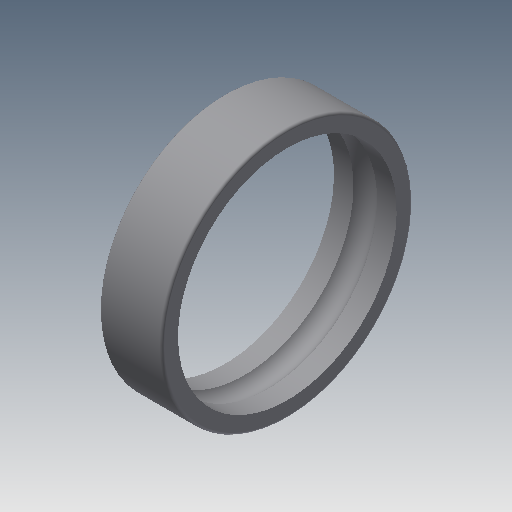
# Autodesk Inventor part: 676A Outer ring
Saved by Autodesk Inventor 2019.4 (Build 234330000, 330)
## iProperties
Category: PARTsolutions
Company: NTN
Created: 2019-06-11
Part Number: 676A Outer ring
Material: 一般
Catalog Web Link: www.cadenas.de
Description: Six types or-Metric system sizes
Vendor: NTN
Document SubType Name: Modeling
Designer: psadmin
Manufacturer: NTN
Mass: 0.0426535 g
Surface Area: 1.86998 cm^2
Volume: 0.0426535 cm^3
Density: 1 g/cm^3
Appearance: PSOLRGB-192-192-192
PSOL_IDENT_0: {$CADENAS_DATA\23d-libs\ntn\ball_roller_bearings\miniature_extra_small_bb\metric_system_sizes\mss_or
PSOL_IDENT_1: .prj},178 {VTYP=3D},{NB=676A Outer ring},{LINA=676A Outer ring},{NN=Six types or},{DATE=29.01.2019 2
PSOL_IDENT_2: 3:03:33},{GEOMDATE=02.04.2007 00:00:00},{VERSION=},{LINEID=9710},{WBVAR=},{WBNUMERIC=}  {NB=676A Out
PSOL_IDENT_3: er ring},{LINA=676A Outer ring},{KT=DUMMY},{IDNR=},{SD=6.0},{D=10},{B=2.5},{R=0.10},{ORDER=676A},{CR=
PSOL_IDENT_4: 465},{COR=196},{CRF=47},{CORF=20},{LSG=43 000},{LSO=51 000},{MASS=0.65},{D1=11.2},{D2=11.2},{C1=0.6}
PSOL_IDENT_5: ,{C2=0.6},{ORDER1=676A},{WSS=WA676AZ},{WDS=ZZ},{UTWF=FL676A},{FORSS=FLWA676AZ},{FORDS=ZZ},{DA1=6,6},
PSOL_IDENT_6: {DA2=6,7},{DA=9,2},{RAS=0,1},{MASS1=0.74},{B1=3.0},{VERS=1},{X=2},{N=12},{O=25.12},{RB=0.592}
NN: Six types or
NT: Metric system sizes
NB: 676A Outer ring
NBSYN: $ORDER. Outer ring
LINA: 676A Outer ring
SD: 6
D: 10
B: 2.5
R: 0.1
CR: 465
COR: 196
CRF: 47
CORF: 20
LSG: 43 000
LSO: 51 000
MASS: 0.65
D1: 11.2
D2: 11.2
C1: 0.6
C2: 0.6
ORDER1: 676A
WSS: WA676AZ
WDS: ZZ
UTWF: FL676A
FORSS: FLWA676AZ
FORDS: ZZ
DA1: 6,6
DA2: 6,7
DA: 9,2
RAS: 0,1
MASS1: 0.74
B1: 3
VERS: 1
SUPPLIER: NTN
ARTICLENO: 676A Outer ring
BOMINFO: 676A Outer ring
CREATOR: CADENAS GmbH
Title: 676A Outer ring
Author: Cadenas PARTsolutions
Comments: Metric system sizes
Autodesk Inventor part; units mm, degrees
sketch "Sketch_1" plane through (0, 0, 0) normal (0, 0, 1) x (1, 0, 0)
  line L0 (2.5, 0) -> (0, 0)
  line L1 (0, 4.9) -> (0, 4.36)
  line L2 (0, 4.36) -> (0.78, 4.36)
  arc A0 (1.72, 4.36) -> (0.78, 4.36) centre (1.25, 4) ccw
  line L3 (1.72, 4.36) -> (2.5, 4.36)
  line L4 (2.5, 4.36) -> (2.5, 4.9)
  arc A1 (2.5, 4.9) -> (2.4, 5) centre (2.4, 4.9) ccw
  line L5 (2.4, 5) -> (0.1, 5)
  arc A2 (0.1, 5) -> (0, 4.9) centre (0.1, 4.9) ccw
  constraints: 12 end point, 6 point on circle, 3 centre point
revolve "Revolution1" add sketch "Sketch_1" angle 360 about axis through (2.5, 0, 0) along (1, 0, 0)
ref_plane "mss_or_XY" through (0, 0, 0) normal (1, 0, 0) x (0, 0, -1)
ref_plane "mss_or_YZ" through (0, 0, 0) normal (0, 0, -1) x (0, 1, 0)
ref_plane "mss_or_ZX" through (0, 0, 0) normal (0, 1, 0) x (1, 0, 0)
ref_plane "mss_or11_XY" through (3, 0, 0) normal (1, 0, 0) x (0, 0, -1)
ref_plane "mss_or11_YZ" through (3, 0, 0) normal (0, 0, -1) x (0, 1, 0)
ref_plane "mss_or11_ZX" through (3, 0, 0) normal (0, 1, 0) x (1, 0, 0)
ref_plane "mss_or2_1_XY" through (1.25, 4, 0) normal (1, 0, 0) x (0, 0, -1)
ref_plane "mss_or2_1_YZ" through (1.25, 4, 0) normal (0, 0, -1) x (0, 1, 0)
ref_plane "mss_or2_1_ZX" through (1.25, 4, 0) normal (0, 1, 0) x (1, 0, 0)
ref_plane "mss_or2_10_XY" through (1.25, 0, -4) normal (1, 0, 0) x (0, 0, -1)
ref_plane "mss_or2_10_YZ" through (1.25, 0, -4) normal (0, 0, -1) x (0, 1, 0)
ref_plane "mss_or2_10_ZX" through (1.25, 0, -4) normal (0, 1, 0) x (1, 0, 0)
ref_plane "mss_or2_11_XY" through (1.25, 2, -3.4641) normal (1, 0, 0) x (0, 0, -1)
ref_plane "mss_or2_11_YZ" through (1.25, 2, -3.4641) normal (0, 0, -1) x (0, 1, 0)
ref_plane "mss_or2_11_ZX" through (1.25, 2, -3.4641) normal (0, 1, 0) x (1, 0, 0)
ref_plane "mss_or2_12_XY" through (1.25, 3.4641, -2) normal (1, 0, 0) x (0, 0, -1)
ref_plane "mss_or2_12_YZ" through (1.25, 3.4641, -2) normal (0, 0, -1) x (0, 1, 0)
ref_plane "mss_or2_12_ZX" through (1.25, 3.4641, -2) normal (0, 1, 0) x (1, 0, 0)
ref_plane "mss_or2_2_XY" through (1.25, 3.4641, 2) normal (1, 0, 0) x (0, 0, -1)
ref_plane "mss_or2_2_YZ" through (1.25, 3.4641, 2) normal (0, 0, -1) x (0, 1, 0)
ref_plane "mss_or2_2_ZX" through (1.25, 3.4641, 2) normal (0, 1, 0) x (1, 0, 0)
ref_plane "mss_or2_3_XY" through (1.25, 2, 3.4641) normal (1, 0, 0) x (0, 0, -1)
ref_plane "mss_or2_3_YZ" through (1.25, 2, 3.4641) normal (0, 0, -1) x (0, 1, 0)
ref_plane "mss_or2_3_ZX" through (1.25, 2, 3.4641) normal (0, 1, 0) x (1, 0, 0)
ref_plane "mss_or2_4_XY" through (1.25, 0, 4) normal (1, 0, 0) x (0, 0, -1)
ref_plane "mss_or2_4_YZ" through (1.25, 0, 4) normal (0, 0, -1) x (0, 1, 0)
ref_plane "mss_or2_4_ZX" through (1.25, 0, 4) normal (0, 1, 0) x (1, 0, 0)
ref_plane "mss_or2_5_XY" through (1.25, -2, 3.4641) normal (1, 0, 0) x (0, 0, -1)
ref_plane "mss_or2_5_YZ" through (1.25, -2, 3.4641) normal (0, 0, -1) x (0, 1, 0)
ref_plane "mss_or2_5_ZX" through (1.25, -2, 3.4641) normal (0, 1, 0) x (1, 0, 0)
ref_plane "mss_or2_6_XY" through (1.25, -3.4641, 2) normal (1, 0, 0) x (0, 0, -1)
ref_plane "mss_or2_6_YZ" through (1.25, -3.4641, 2) normal (0, 0, -1) x (0, 1, 0)
ref_plane "mss_or2_6_ZX" through (1.25, -3.4641, 2) normal (0, 1, 0) x (1, 0, 0)
ref_plane "mss_or2_7_XY" through (1.25, -4, 0) normal (1, 0, 0) x (0, 0, -1)
ref_plane "mss_or2_7_YZ" through (1.25, -4, 0) normal (0, 0, -1) x (0, 1, 0)
ref_plane "mss_or2_7_ZX" through (1.25, -4, 0) normal (0, 1, 0) x (1, 0, 0)
ref_plane "mss_or2_8_XY" through (1.25, -3.4641, -2) normal (1, 0, 0) x (0, 0, -1)
ref_plane "mss_or2_8_YZ" through (1.25, -3.4641, -2) normal (0, 0, -1) x (0, 1, 0)
ref_plane "mss_or2_8_ZX" through (1.25, -3.4641, -2) normal (0, 1, 0) x (1, 0, 0)
ref_plane "mss_or2_9_XY" through (1.25, -2, -3.4641) normal (1, 0, 0) x (0, 0, -1)
ref_plane "mss_or2_9_YZ" through (1.25, -2, -3.4641) normal (0, 0, -1) x (0, 1, 0)
ref_plane "mss_or2_9_ZX" through (1.25, -2, -3.4641) normal (0, 1, 0) x (1, 0, 0)
ref_plane "mss_or21_1_XY" through (1.5, 4, 0) normal (1, 0, 0) x (0, 0, -1)
ref_plane "mss_or21_1_YZ" through (1.5, 4, 0) normal (0, 0, -1) x (0, 1, 0)
ref_plane "mss_or21_1_ZX" through (1.5, 4, 0) normal (0, 1, 0) x (1, 0, 0)
ref_plane "mss_or21_10_XY" through (1.5, 0, -4) normal (1, 0, 0) x (0, 0, -1)
ref_plane "mss_or21_10_YZ" through (1.5, 0, -4) normal (0, 0, -1) x (0, 1, 0)
ref_plane "mss_or21_10_ZX" through (1.5, 0, -4) normal (0, 1, 0) x (1, 0, 0)
ref_plane "mss_or21_11_XY" through (1.5, 2, -3.4641) normal (1, 0, 0) x (0, 0, -1)
ref_plane "mss_or21_11_YZ" through (1.5, 2, -3.4641) normal (0, 0, -1) x (0, 1, 0)
ref_plane "mss_or21_11_ZX" through (1.5, 2, -3.4641) normal (0, 1, 0) x (1, 0, 0)
ref_plane "mss_or21_12_XY" through (1.5, 3.4641, -2) normal (1, 0, 0) x (0, 0, -1)
ref_plane "mss_or21_12_YZ" through (1.5, 3.4641, -2) normal (0, 0, -1) x (0, 1, 0)
ref_plane "mss_or21_12_ZX" through (1.5, 3.4641, -2) normal (0, 1, 0) x (1, 0, 0)
ref_plane "mss_or21_2_XY" through (1.5, 3.4641, 2) normal (1, 0, 0) x (0, 0, -1)
ref_plane "mss_or21_2_YZ" through (1.5, 3.4641, 2) normal (0, 0, -1) x (0, 1, 0)
ref_plane "mss_or21_2_ZX" through (1.5, 3.4641, 2) normal (0, 1, 0) x (1, 0, 0)
ref_plane "mss_or21_3_XY" through (1.5, 2, 3.4641) normal (1, 0, 0) x (0, 0, -1)
ref_plane "mss_or21_3_YZ" through (1.5, 2, 3.4641) normal (0, 0, -1) x (0, 1, 0)
ref_plane "mss_or21_3_ZX" through (1.5, 2, 3.4641) normal (0, 1, 0) x (1, 0, 0)
ref_plane "mss_or21_4_XY" through (1.5, 0, 4) normal (1, 0, 0) x (0, 0, -1)
ref_plane "mss_or21_4_YZ" through (1.5, 0, 4) normal (0, 0, -1) x (0, 1, 0)
ref_plane "mss_or21_4_ZX" through (1.5, 0, 4) normal (0, 1, 0) x (1, 0, 0)
ref_plane "mss_or21_5_XY" through (1.5, -2, 3.4641) normal (1, 0, 0) x (0, 0, -1)
ref_plane "mss_or21_5_YZ" through (1.5, -2, 3.4641) normal (0, 0, -1) x (0, 1, 0)
ref_plane "mss_or21_5_ZX" through (1.5, -2, 3.4641) normal (0, 1, 0) x (1, 0, 0)
ref_plane "mss_or21_6_XY" through (1.5, -3.4641, 2) normal (1, 0, 0) x (0, 0, -1)
ref_plane "mss_or21_6_YZ" through (1.5, -3.4641, 2) normal (0, 0, -1) x (0, 1, 0)
ref_plane "mss_or21_6_ZX" through (1.5, -3.4641, 2) normal (0, 1, 0) x (1, 0, 0)
ref_plane "mss_or21_7_XY" through (1.5, -4, 0) normal (1, 0, 0) x (0, 0, -1)
ref_plane "mss_or21_7_YZ" through (1.5, -4, 0) normal (0, 0, -1) x (0, 1, 0)
ref_plane "mss_or21_7_ZX" through (1.5, -4, 0) normal (0, 1, 0) x (1, 0, 0)
ref_plane "mss_or21_8_XY" through (1.5, -3.4641, -2) normal (1, 0, 0) x (0, 0, -1)
ref_plane "mss_or21_8_YZ" through (1.5, -3.4641, -2) normal (0, 0, -1) x (0, 1, 0)
ref_plane "mss_or21_8_ZX" through (1.5, -3.4641, -2) normal (0, 1, 0) x (1, 0, 0)
ref_plane "mss_or21_9_XY" through (1.5, -2, -3.4641) normal (1, 0, 0) x (0, 0, -1)
ref_plane "mss_or21_9_YZ" through (1.5, -2, -3.4641) normal (0, 0, -1) x (0, 1, 0)
ref_plane "mss_or21_9_ZX" through (1.5, -2, -3.4641) normal (0, 1, 0) x (1, 0, 0)
body "Solid1"
